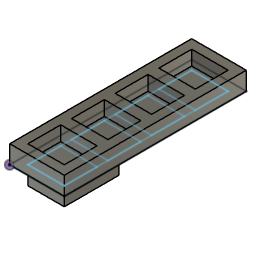
Compartment Archive (Autodesk Fusion 360 design; units mm, degrees)
Autodesk Fusion 360 part; units mm, degrees
sketch " Compartment Divet" plane through (0, 0, 0) normal (0, 0, 1) x (1, 0, 0)
  line L0 (5, 5) -> (25, 5) construction
  line L1 (25, 5) -> (25, 35) construction
  line L2 (25, 35) -> (5, 35) construction
  line L3 (5, 35) -> (5, 5) construction
  line L4 (5, 35) -> (25, 35)
  line L5 (25, 35) -> (25, 5)
  line L6 (25, 5) -> (5, 5)
  line L7 (5, 5) -> (5, 35)
  dimension "d3" = 20
  dimension "d4" = 30
  constraint horizontal L0
  constraint vertical L1
  constraint horizontal L2
  constraint vertical L3
  constraint horizontal L4
  constraint vertical L5
  constraint horizontal L6
  constraint vertical L7
  measures "d3" distance of L0.start L0.end
  measures "d4" distance of L0.start L2.end
sketch "Compartment Body" plane through (0, 0, 0) normal (0, 0, 1) x (1, 0, 0)
  line L0 (0, 0) -> (30, 0)
  line L1 (30, 0) -> (30, 100)
  line L2 (30, 100) -> (0, 100)
  line L3 (0, 100) -> (0, 0)
  line L4 (5, 95) -> (25, 95)
  line L5 (25, 95) -> (25, 5)
  line L6 (25, 5) -> (5, 5)
  line L7 (5, 5) -> (5, 95)
  line L8 (5, 95) -> (25, 95)
  line L9 (25, 95) -> (25, 77)
  line L10 (25, 77) -> (5, 77)
  line L11 (5, 77) -> (5, 95)
  line L12 (5, 71) -> (25, 71)
  line L13 (25, 71) -> (25, 53)
  line L14 (25, 53) -> (5, 53)
  line L15 (5, 53) -> (5, 71)
  line L16 (5, 47) -> (25, 47)
  line L17 (25, 47) -> (25, 29)
  line L18 (25, 29) -> (5, 29)
  line L19 (5, 29) -> (5, 47)
  line L20 (5, 23) -> (25, 23)
  line L21 (25, 23) -> (25, 5)
  line L22 (25, 5) -> (5, 5)
  line L23 (5, 5) -> (5, 23)
  dimension "d7" = 30
  dimension "d8" = 100
  dimension "d11" = 18
  dimension "d12" = 18
  dimension "d13" = 18
  dimension "d14" = 18
  constraint horizontal L0
  constraint vertical L1
  constraint horizontal L2
  constraint vertical L3
  constraint coincident L0.start L3.end
  constraint horizontal L4
  constraint vertical L5
  constraint horizontal L6
  constraint vertical L7
  constraint horizontal L8
  constraint vertical L9
  constraint horizontal L10
  constraint vertical L11
  constraint horizontal L12
  constraint vertical L13
  constraint horizontal L14
  constraint vertical L15
  constraint horizontal L16
  constraint vertical L17
  constraint horizontal L18
  constraint vertical L19
  constraint horizontal L20
  constraint vertical L21
  constraint horizontal L22
  constraint vertical L23
  measures "d7" distance of L0.start L0.end
  measures "d8" distance of L0.start L2.end
  measures "d11" distance of L4.start L10.end
  measures "d12" distance of L12.start L14.end
  measures "d13" distance of L18.end L16.start
  measures "d14" distance of L20.start L6.end
extrude "Extrude2" add sketch " Compartment Divet" against normal blind 10 makes body 1
extrude "Extrude3" add sketch "Compartment Body" along normal blind 5 contours L4 L5 L7 L8 L9 L10 L11 | L5 L7 L12 L13 L14 L15 | L5 L7 L16 L17 L18 L19 | L5 L6 L7 L20 L21 L22 L23 bodies 1 makes body 2 at (11.6667, 65, 0) makes body 3 at (11.6667, 89, 0)
extrude "Extrude4" add sketch "Compartment Body" along normal blind 10 contours L0 L1 L2 L3 | L5 L7 L10 L12 | L5 L7 L14 L16 | L5 L7 L18 L20 bodies 1 2 3
extrude "Extrude5" cut 4 faces at (11.6667, 17, 5) (18.3333, 41, 5) (11.6667, 65, 5) (11.6667, 89, 5) along direction (0, 0, -1) blind 3 on bodies 1 bodies 1
